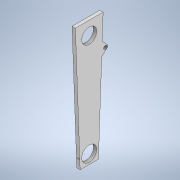
# Autodesk Inventor part: Intake - Side Panel
Saved by Autodesk Inventor 2020 (Build 240168000, 168)
## iProperties
Created: 2020-02-06
Part Number: Intake - Side Panel
Material: Generic
Document SubType Name: Modeling
Designer: aidan
Density: 1 g/cm^3
Appearance: Default
Author: aidan
Autodesk Inventor part; units mm, degrees
ref_plane "YZ Plane" through (0, 0, 0) normal (1, 0, 0) x (0, 1, 0)
ref_plane "XZ Plane" through (0, 0, 0) normal (0, 1, 0) x (-1, 0, 0)
ref_plane "XY Plane" through (0, 0, 0) normal (0, 0, 1) x (1, 0, 0)
sketch "Sketch1" plane through (0, 0, 0) normal (1, 0, 0) x (0, 1, 0)
  line L0 (0, -38.1) -> (169.0878, -44.45)
  line L1 (169.0878, -44.45) -> (169.0878, 6.35)
  line L2 (169.0878, 6.35) -> (0, 0)
  line L3 (0, 0) -> (0, -38.1)
  arc A0 (169.0878, -44.45) -> (169.0878, 6.35) centre (169.0878, -19.05) ccw
  circle A1 centre (169.0878, -19.05) radius 14.2875
  point P0 (0, -19.05)
  point P1 (169.0878, -33.3375)
  point P2 (169.0878, -4.7625)
  dimension "d3" = 50.8
  dimension "d4" = 38.1
  dimension "d5" = 28.575
  dimension "d9" = 169.0878
  constraints: 8 end point, 3 coincident, 3 point on circle, 2 centre point, 2 midpoint, 1 horizontal alignment, 1 parallel, 1 point on line, 1 vertical
  measures "d3" distance of L0.end L1.end
  measures "d4" distance of L0.start L2.end
  measures "d5" diameter of A1
  measures "d9" distance between parallel lines of L3 L1
extrude "Extrusion1" add sketch "Sketch1" against normal blind 6.35 contours L3 L2 L1 A1 L0 | L1 A1 A0
sketch "Sketch3" plane through (-6.35, 0, 0) normal (-1, 0, 0) x (0, 0, 1)
  line L0 (-38.1, 0) -> (0, 0) projected
  line L1 (0, 0) -> (-0.9539, -25.4)
  line L2 (-44.45, 169.0878) -> (-38.1, 0) projected
  line L3 (-38.1, 0) -> (-37.1461, -25.4)
  line L4 (0, 0) -> (6.35, 169.0878) projected
  line L5 (-37.1461, -25.4) -> (-0.9539, -25.4)
  arc A0 (-37.1461, -25.4) -> (-0.9539, -25.4) centre (-19.05, -25.4) ccw
  circle A1 centre (-19.05, -25.4) radius 14.2875
  dimension "d12" = 25.4
  dimension "d13" = 28.575
  constraints: 6 end point, 2 centre point, 2 collinear, 2 point on circle, 1 coincident, 1 midpoint, 1 parallel
  measures "d12" distance between parallel lines of L0 L5
  measures "d13" diameter of A1
extrude "Extrusion2" add sketch "Sketch3" against normal blind 6.35 contours L0 L1 L5 A1 L3 | L5 A1 A0
sketch "Sketch4" plane through (-6.35, 0, 0) normal (-1, 0, 0) x (0, 0, 1)
  line L0 (6.35, 169.0878) -> (-0.9539, -25.4) projected
  line L1 (-0.9539, -25.4) -> (-1.6335, -43.4961)
  line L2 (-37.1461, -25.4) -> (-44.45, 169.0878) projected
  line L3 (-37.1461, -25.4) -> (-36.4665, -43.4961)
  arc A0 (-37.1461, -25.4) -> (-0.9539, -25.4) centre (-19.05, -25.4) ccw projected
  line L4 (-1.6335, -43.4961) -> (-36.4665, -43.4961)
  line L5 (6.35, 169.0878) -> (7.3039, 194.4878)
  line L6 (-44.45, 169.0878) -> (-45.4039, 194.4878)
  arc A1 (6.35, 169.0878) -> (-44.45, 169.0878) centre (-19.05, 169.0878) ccw projected
  line L7 (7.3039, 194.4878) -> (-45.4039, 194.4878)
  point P0 (0, 0)
  point P1 (-19.05, -43.4961)
  point P2 (-19.05, -43.4961)
  point P3 (-19.05, 194.4878)
  point P4 (-19.05, 194.4878)
  point P5 (-19.05, -43.4961)
  point P6 (-1.0049, -26.7573)
  point P7 (-37.0951, -26.7573)
  point P8 (-19.05, 194.4878)
  constraints: 12 end point, 4 collinear, 4 horizontal alignment, 4 point on circle, 2 horizontal
extrude "Extrusion3" add sketch "Sketch4" against normal blind 6.35 contours A1 L7 L5 | A1 L6 L7 | L1 L4 A0 | L4 L3 A0
sketch "Sketch5" plane through (-6.35, 0, 0) normal (-1, 0, 0) x (0, 0, 1)
  circle A0 centre (-49.5027, 134.3039) radius 3.175
  line L0 (-36.4665, -43.4961) -> (-1.6335, -43.4961) projected
  line L1 (-0.9539, -25.4) -> (7.3039, 194.4878) projected
  line L2 (-45.4039, 194.4878) -> (-37.1461, -25.4) projected
  line L3 (-43.6385, 147.4805) -> (-55.8527, 134.3039)
  line L4 (-55.8527, 134.3039) -> (-42.6847, 122.0805)
  point P0 (0, 0)
  dimension "d18" = 6.35
  dimension "d19" = 177.8
  dimension "d29" = 25.4
  dimension "d30" = 12.7
  dimension "d31" = 6.35
  constraints: 4 end point, 2 point on line, 1 centre point, 1 equal length, 1 horizontal alignment
  measures "d18" diameter of A0
  measures "d19" distance from line of L0 A0.centre
  measures "d29" vertical distance of L4.end L3.start
  measures "d30" distance from line of L3.end L2
  measures "d31" distance of L3.end A0.centre
extrude "Extrusion4" add sketch "Sketch5" against normal blind 6.35
fillet "Fillet1" radius 3.175 1 edges at (-3.175, 134.3039, -55.8527)
body "Solid1"
